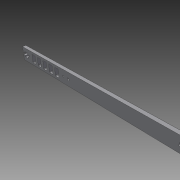
# Autodesk Inventor part: front_pane_middle
Saved by Autodesk Inventor 2014 (Build 180170000, 170)
## iProperties
Created: 2014-03-23
Part Number: front_pane_middle
Material: Plywood, Finish
Document SubType Name: Modeling
Designer: buben
Density: 0.552 g/cm^3
Appearance: Plywood - New
Author: buben
Autodesk Inventor part; units mm, degrees
ref_plane "YZ Plane" through (0, 0, 0) normal (1, 0, 0) x (0, 1, 0)
ref_plane "XZ Plane" through (0, 0, 0) normal (0, 1, 0) x (-1, 0, 0)
ref_plane "XY Plane" through (0, 0, 0) normal (0, 0, 1) x (1, 0, 0)
sketch "Sketch1" plane through (0, 0, 0) normal (0, 1, 0) x (-1, 0, 0)
  line L0 (0, 0) -> (-300, 0)
  line L1 (-300, 0) -> (-300, -23.685)
  line L2 (-300, -23.685) -> (0, -23.685)
  line L3 (0, -23.685) -> (0, 0)
  dimension "d0" = 300
  dimension "d1" = 23.685
  constraints: 8 end point, 2 parallel, 1 horizontal, 1 perpendicular
  measures "d0" distance of L0.start L0.end
  measures "d1" distance of L2.end L0.start
extrude "Extrusion1" add sketch "Sketch1" along normal blind 6.5
sketch "Sketch2" plane through (0, 6.5, 0) normal (0, 1, 0) x (1, 0, 0)
  line L0 (0, 23.685) -> (0, 0) projected
  line L1 (26, 19.3425) -> (32, 19.3425)
  line L2 (33, 18.3425) -> (33, 5.3425)
  line L3 (32, 4.3425) -> (26, 4.3425)
  line L4 (25, 5.3425) -> (25, 18.3425)
  arc A0 (26, 19.3425) -> (25, 18.3425) centre (26, 18.3425) ccw
  arc A1 (25, 5.3425) -> (26, 4.3425) centre (26, 5.3425) ccw
  arc A2 (32, 4.3425) -> (33, 5.3425) centre (32, 5.3425) ccw
  arc A3 (33, 18.3425) -> (32, 19.3425) centre (32, 18.3425) ccw
  point P0 (25, 11.8425)
  point P1 (0, 11.8425)
  dimension "d4" = 1
  dimension "d5" = 15
  dimension "d6" = 8
  dimension "d7" = 25
  constraints: 8 end point, 8 point on circle, 8 tangent, 4 centre point, 3 equal radius, 2 midpoint, 2 parallel, 1 horizontal, 1 horizontal alignment, 1 perpendicular
  measures "d4" radius of A0
  measures "d5" distance between parallel lines of L3 L1
  measures "d6" distance between parallel lines of L2 L4
  measures "d7" distance between parallel lines of L0 L4
extrude "Extrusion2" cut sketch "Sketch2" against normal through all
pattern_linear "Rectangular Pattern1" count 5 spacing 14 along (1, 0, 0) of "Extrusion2"
sketch "Sketch3" plane through (0, 0, 0) normal (0, -1, 0) x (1, 0, 0)
  line L0 (0, 0) -> (300, 0) projected
  line L1 (0, -23.685) -> (0, 0) projected
  line L2 (300, -23.685) -> (0, -23.685) projected
  line L3 (16.3, -9.5925) -> (16.3, -14.0925)
  line L4 (0, -14.0925) -> (0, -9.5925)
  line L5 (5, -7.0925) -> (12.3, -7.0925)
  line L6 (12.3, -16.5925) -> (5, -16.5925)
  line L7 (150, 0) -> (150, -23.685) construction
  line L8 (0, -9.5925) -> (5, -9.5925)
  line L9 (12.3, -9.5925) -> (16.3, -9.5925)
  line L10 (16.3, -14.0925) -> (12.3, -14.0925)
  line L11 (5, -14.0925) -> (0, -14.0925)
  line L12 (5, -16.5925) -> (5, -14.0925)
  line L13 (5, -9.5925) -> (5, -7.0925)
  line L14 (12.3, -7.0925) -> (12.3, -9.5925)
  line L15 (12.3, -14.0925) -> (12.3, -16.5925)
  line L16 (283.7, -9.5925) -> (283.7, -14.0925)
  line L17 (300, -14.0925) -> (300, -9.5925)
  line L18 (295, -7.0925) -> (287.7, -7.0925)
  line L19 (287.7, -16.5925) -> (295, -16.5925)
  line L20 (300, -9.5925) -> (295, -9.5925)
  line L21 (287.7, -9.5925) -> (283.7, -9.5925)
  line L22 (283.7, -14.0925) -> (287.7, -14.0925)
  line L23 (295, -14.0925) -> (300, -14.0925)
  line L24 (295, -16.5925) -> (295, -14.0925)
  line L25 (295, -9.5925) -> (295, -7.0925)
  line L26 (287.7, -7.0925) -> (287.7, -9.5925)
  line L27 (287.7, -14.0925) -> (287.7, -16.5925)
  point P0 (16.3, -11.8425)
  point P1 (0, -11.8425)
  point P2 (283.7, -11.8425)
  point P3 (300, -11.8425)
  dimension "d13" = 4.5
  dimension "d14" = 5
  dimension "d15" = 4
  dimension "d16" = 7.3
  dimension "d17" = 2.5
  constraints: 50 end point, 14 symmetric about line, 10 parallel, 6 collinear, 4 midpoint, 4 perpendicular, 3 horizontal, 1 horizontal alignment
  measures "d13" distance of L3.start L3.end
  measures "d14" distance of L4.end L8.end
  measures "d15" distance of L9.start L3.start
  measures "d16" distance of L5.start L5.end
  measures "d17" distance of L8.end L5.start
extrude "Extrusion3" cut sketch "Sketch3" against normal through all
sketch "Sketch4" plane through (0, 6.5, 0) normal (0, 1, 0) x (1, 0, 0)
  line L0 (16.3, 14.0925) -> (16.3, 9.5925) projected
  line L1 (0, 9.5925) -> (0, 0) projected
  line L2 (89, 18.3425) -> (89, 5.3425) projected
  circle A0 centre (110, 11.8425) radius 2.25
  circle A1 centre (99, 11.8425) radius 1.5
  point P0 (16.3, 11.8425)
  dimension "d20" = 110
  dimension "d21" = 4.5
  dimension "d22" = 3
  dimension "d23" = 10
  constraints: 2 centre point, 2 horizontal alignment, 1 midpoint
  measures "d20" distance from line of L1 A0.centre
  measures "d21" diameter of A0
  measures "d22" diameter of A1
  measures "d23" distance from line of L2 A1.centre
extrude "Extrusion4" cut sketch "Sketch4" against normal through all
body "Solid1"
